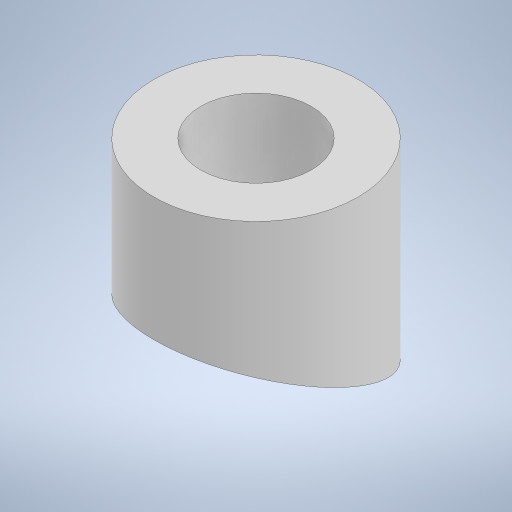
# Autodesk Inventor part: Test - 16.25mmID at 22.4degAngle
Saved by Autodesk Inventor 2023 (Build 270158000, 158)
## iProperties
Created: 2023-01-23
Part Number: Test - 16.25mmID at 22.4degAngle
Material: Generic
Document SubType Name: Modeling
Designer: Administrator
Density: 1 g/cm^3
Appearance: Default
Author: Administrator
Autodesk Inventor part; units mm, degrees
ref_plane "YZ Plane" through (0, 0, 0) normal (1, 0, 0) x (0, 1, 0)
ref_plane "XZ Plane" through (0, 0, 0) normal (0, 1, 0) x (-1, 0, 0)
ref_plane "XY Plane" through (0, 0, 0) normal (0, 0, 1) x (1, 0, 0)
sketch "Sketch1" plane through (0, 0, 0) normal (0, 1, 0) x (-1, 0, 0)
  circle A0 centre (0, 0) radius 15
  circle A1 centre (0, 0) radius 8.125
  line L0 (20.2243, -15) -> (-24.2089, -15) construction
  dimension "d0" = 30
  dimension "d1" = 16.25
  constraints: 2 centre point, 2 coincident, 2 end point, 1 horizontal, 1 tangent
  measures "d0" diameter of A0
  measures "d1" diameter of A1
extrude "Extrusion1" add sketch "Sketch1" along normal blind 30
ref_plane "Work Plane1" through (-20.2243, 0, -15) normal (0, -0.9304176, 0.3665012) x (1, 0, 0)
sketch "Sketch2" plane through (-20.2243, 0, -15) normal (0, -0.9304176, 0.3665012) x (1, 0, 0)
  line L0 (1.1433, -5.018) -> (38.442, -5.018)
  line L1 (38.442, -5.018) -> (38.442, 42.5884)
  line L2 (38.442, 42.5884) -> (1.1433, 42.5884)
  line L3 (1.1433, 42.5884) -> (1.1433, -5.018)
  point P0 (20.2243, 13.9563)
  constraints: 8 end point, 2 parallel, 1 horizontal, 1 perpendicular
extrude "Extrusion2" cut sketch "Sketch2" along normal blind 20
body "Solid1"
